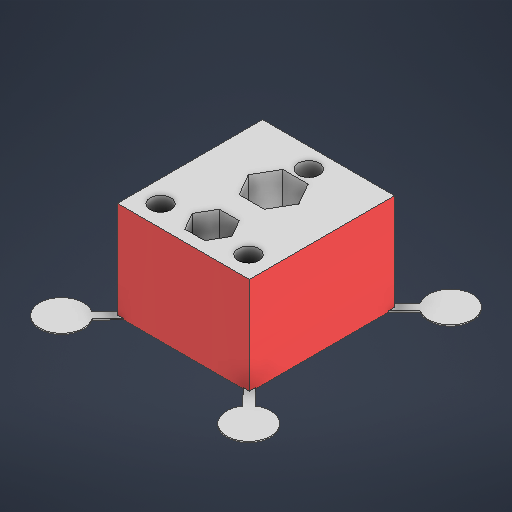
# Autodesk Inventor part: adapter-optical
Saved by Autodesk Inventor 2026.2 (Build 302298000, 298)
## iProperties
Created: 2026-05-22
Part Number: adapter-optical
Material: Generic
Document SubType Name: Modeling
Designer: mayhe
Density: 1 g/cm^3
Appearance: Default
Author: mayhe
Autodesk Inventor part; units mm, degrees
ref_plane "YZ Plane" through (0, 0, 0) normal (1, 0, 0) x (0, 1, 0)
ref_plane "XZ Plane" through (0, 0, 0) normal (0, 1, 0) x (-1, 0, 0)
ref_plane "XY Plane" through (0, 0, 0) normal (0, 0, 1) x (1, 0, 0)
sketch "Sketch1" plane through (0, 0, 0) normal (1, 0, 0) x (0, 1, 0)
  line L0 (11.125, 16.5) -> (-11.125, 16.5)
  line L1 (-11.125, 16.5) -> (-11.125, -16.5)
  line L2 (-11.125, -16.5) -> (11.125, -16.5)
  line L3 (11.125, -16.5) -> (11.125, 16.5)
  line L4 (11.125, 16.5) -> (-11.125, -16.5) construction
  line L5 (-11.125, 16.5) -> (11.125, -16.5) construction
  point P0 (0, 0)
  dimension "d0" = 22.25
  dimension "d1" = 33
  constraints: 12 end point, 2 midpoint, 2 parallel, 1 horizontal, 1 perpendicular
  measures "d0" distance of L2.end L1.end
  measures "d1" distance of L1.end L0.end
extrude "Extrusion1" add sketch "Sketch1" along normal mid plane 30
sketch "Sketch2" plane through (-15, -11.125, -16.5) normal (0, -1, 0) x (1, 0, 0)
  circle A0 centre (15, 4.5) radius 2.25
  line L0 (0, 0) -> (30, 0) projected
  circle A1 centre (25, 28.2) radius 2.25
  circle A2 centre (5, 28.2) radius 2.25
  point P0 (15, 16.5)
  dimension "d4" = 4.5
  dimension "d5" = 4.5
  dimension "d6" = 4.5
  dimension "d7" = 4.5
  dimension "d8" = 23.7
  dimension "d9" = 10
  dimension "d10" = 10
  constraints: 3 centre point, 1 horizontal alignment
  measures "d4" diameter of A0
  measures "d5" distance from line of L0 A0.centre
  measures "d6" diameter of A1
  measures "d7" diameter of A2
  measures "d8" vertical distance of A1.centre A0.centre
  measures "d9" horizontal distance of A0.centre A1.centre
  measures "d10" horizontal distance of A2.centre A0.centre
hole "Hole1" at (0, -11.125, -12) at (-10, -11.125, 11.7) at (10, -11.125, 11.7) direction (0, 1, 0) diameter 4.75 depth 22.25 tip angle 118 counterbore diameter 7.5 counterbore depth 3
sketch "Sketch4" plane through (-15, -11.125, -16.5) normal (0, -1, 0) x (1, 0, 0)
  circle A0 centre (15, 12.5) radius 2.0256
  circle A1 centre (15, 26.5) radius 2.1001
  line L0 (30, 33) -> (0, 33) projected
  point P0 (15, 16.5)
  point P1 (15, 33)
  dimension "d23" = 14
  dimension "d24" = 6.5
  constraints: 2 centre point, 1 midpoint
  measures "d23" distance of A1.centre A0.centre
  measures "d24" distance of point (15, 33) A1.centre
hole "Big Hole" at (0, -11.125, -4) direction (0, 1, 0) diameter 6.75 depth 22.25 tip angle 118
hole "Small Hole1" at (0, -11.125, 10) direction (0, 1, 0) diameter 5.75 depth 22.25 tip angle 118
sketch "Sketch5" plane through (-15, 11.125, 16.5) normal (0, 1, 0) x (1, 0, 0)
  circle A0 centre (15, 6.5) radius 2.875 projected
  circle A1 centre (15, 20.5) radius 3.375 projected
  circle A2 centre (15, 20.5) radius 4.975
  circle A3 centre (15, 6.5) radius 3.925
  line L0 (17.2661, 10.425) -> (19.5322, 6.5)
  line L1 (19.5322, 6.5) -> (17.2661, 2.575)
  line L2 (17.2661, 2.575) -> (12.7339, 2.575)
  line L3 (12.7339, 2.575) -> (10.4678, 6.5)
  line L4 (10.4678, 6.5) -> (12.7339, 10.425)
  line L5 (12.7339, 10.425) -> (17.2661, 10.425)
  line L6 (17.8723, 25.475) -> (20.7446, 20.5)
  line L7 (20.7446, 20.5) -> (17.8723, 15.525)
  line L8 (17.8723, 15.525) -> (12.1277, 15.525)
  line L9 (12.1277, 15.525) -> (9.2554, 20.5)
  line L10 (9.2554, 20.5) -> (12.1277, 25.475)
  line L11 (12.1277, 25.475) -> (17.8723, 25.475)
  point P0 (15, 16.5)
  point P1 (15, 10.425)
  point P2 (15, 25.475)
  dimension "d39" = 9.95
  dimension "d40" = 7.85
  constraints: 24 end point, 4 coincident, 2 midpoint, 2 vertical alignment, 30 other
extrude "Big nut seat" cut sketch "Sketch5" against normal blind 8.1168 contours A1 | A2 | A2 L6 L7 | A2 L11 L6 | L7 L8 A2 | A2 L10 L11 | L8 L9 A2 | A2 L9 L10
extrude "small nut seat" cut sketch "Sketch5" against normal blind 6.6168 contours A0 | A3 | A3 L0 L1 | A3 L5 L0 | L1 L2 A3 | A3 L4 L5 | L2 L3 A3 | A3 L3 L4
sketch "Sketch6" plane through (15, 11.125, -16.5) normal (0, 0, -1) x (-1, 0, 0)
  line L0 (2.368, -2.6371) -> (27.632, -2.6371) construction
  line L1 (27.632, -2.6371) -> (27.632, -19.6129) construction
  line L2 (27.632, -19.6129) -> (2.368, -19.6129) construction
  line L3 (2.368, -19.6129) -> (2.368, -2.6371) construction
  line L4 (12.625, 0) -> (17.375, 0) projected
  line L5 (15, 0) -> (15, -22.25)
  line L6 (17.875, -22.25) -> (12.125, -22.25) projected
  line L7 (30, 0) -> (0, 0) projected
  spline S0 degree 2 poles (10.4806, -3.0109) (10.4806, -3.7828) (9.6573, -4.6653) (8.942, -4.6653) knots 0 0 0 1 2 2 2
  spline S1 degree 2 poles (8.942, -4.6653) (8.2242, -4.6653) (7.406, -3.7725) (7.406, -3.0109) knots 0 0 0 1 2 2 2
  spline S2 degree 2 poles (7.406, -3.0109) (7.406, -2.2468) (8.2242, -1.3565) (8.942, -1.3565) knots 0 0 0 1 2 2 2
  spline S3 degree 2 poles (8.942, -1.3565) (9.6573, -1.3565) (10.4806, -2.2416) (10.4806, -3.0109) knots 0 0 0 1 2 2 2
  spline S4 degree 2 poles (9.6573, -3.0109) (9.6573, -2.7253) (9.5415, -2.3265) (9.4412, -2.2005) knots 0 0 0 1 2 2 2
  spline S5 degree 2 poles (9.4412, -2.2005) (9.3408, -2.0692) (9.0835, -1.956) (8.9446, -1.956) knots 0 0 0 1 2 2 2
  spline S6 degree 2 poles (8.9446, -1.956) (8.7979, -1.956) (8.5587, -2.0615) (8.448, -2.1953) knots 0 0 0 1 2 2 2
  spline S7 degree 2 poles (8.448, -2.1953) (8.3503, -2.3188) (8.2293, -2.7279) (8.2293, -3.0109) knots 0 0 0 1 2 2 2
  spline S8 degree 2 poles (8.2293, -3.0109) (8.2293, -3.3043) (8.3451, -3.6902) (8.4455, -3.8214) knots 0 0 0 1 2 2 2
  spline S9 degree 2 poles (8.4455, -3.8214) (8.5458, -3.9526) (8.8057, -4.0658) (8.9446, -4.0658) knots 0 0 0 1 2 2 2
  spline S10 degree 2 poles (8.9446, -4.0658) (9.0861, -4.0658) (9.3486, -3.9449) (9.4438, -3.8163) knots 0 0 0 1 2 2 2
  spline S11 degree 2 poles (9.4438, -3.8163) (9.5467, -3.6773) (9.6573, -3.3094) (9.6573, -3.0109) knots 0 0 0 1 2 2 2
  spline S12 degree 2 poles (13.2568, -3.3686) (13.2568, -3.9423) (12.6754, -4.6448) (12.2482, -4.6448) knots 0 0 0 1 2 2 2
  spline S13 degree 2 poles (12.2482, -4.6448) (12.0707, -4.6448) (11.8057, -4.565) (11.6565, -4.4775) knots 0 0 0 1 2 2 2
  line L8 (11.6565, -4.4775) -> (11.6565, -5.4758)
  line L9 (11.6565, -5.4758) -> (10.9103, -5.4758)
  line L10 (10.9103, -5.4758) -> (10.9103, -2.203)
  line L11 (10.9103, -2.203) -> (11.6565, -2.203)
  line L12 (11.6565, -2.203) -> (11.6565, -2.4552)
  spline S14 degree 2 poles (11.6565, -2.4552) (11.8211, -2.3137) (12.1608, -2.1387) (12.3846, -2.1387) knots 0 0 0 1 2 2 2
  spline S15 degree 2 poles (12.3846, -2.1387) (12.8014, -2.1387) (13.2568, -2.8) (13.2568, -3.3686) knots 0 0 0 1 2 2 2
  spline S16 degree 2 poles (12.4927, -3.384) (12.4927, -3.0341) (12.2766, -2.7202) (12.0501, -2.7202) knots 0 0 0 1 2 2 2
  spline S17 degree 2 poles (12.0501, -2.7202) (11.9498, -2.7202) (11.7517, -2.7845) (11.6565, -2.8488) knots 0 0 0 1 2 2 2
  line L13 (11.6565, -2.8488) -> (11.6565, -4.0504)
  spline S18 degree 2 poles (11.6565, -4.0504) (11.7157, -4.0761) (11.8597, -4.0967) (11.9575, -4.0967) knots 0 0 0 1 2 2 2
  spline S19 degree 2 poles (11.9575, -4.0967) (12.2277, -4.0967) (12.4927, -3.7417) (12.4927, -3.384) knots 0 0 0 1 2 2 2
  spline S20 degree 2 poles (14.5742, -4.6448) (14.1188, -4.6448) (13.702, -4.2691) (13.702, -3.842) knots 0 0 0 1 2 2 2
  line L14 (13.702, -3.842) -> (13.702, -2.7228)
  line L15 (13.702, -2.7228) -> (13.4164, -2.7228)
  line L16 (13.4164, -2.7228) -> (13.4164, -2.203)
  line L17 (13.4164, -2.203) -> (13.702, -2.203)
  line L18 (13.702, -2.203) -> (13.702, -1.5186)
  line L19 (13.702, -1.5186) -> (14.4481, -1.5186)
  line L20 (14.4481, -1.5186) -> (14.4481, -2.203)
  line L21 (14.4481, -2.203) -> (15.1685, -2.203)
  line L22 (15.1685, -2.203) -> (15.1685, -2.7228)
  line L23 (15.1685, -2.7228) -> (14.4481, -2.7228)
  line L24 (14.4481, -2.7228) -> (14.4481, -3.5744)
  spline S21 degree 2 poles (14.4481, -3.5744) (14.4481, -3.7005) (14.4533, -3.8883) (14.4841, -3.9629) knots 0 0 0 1 2 2 2
  spline S22 degree 2 poles (14.4841, -3.9629) (14.515, -4.0375) (14.6668, -4.125) (14.8109, -4.125) knots 0 0 0 1 2 2 2
  spline S23 degree 2 poles (14.8109, -4.125) (14.8726, -4.125) (15.0656, -4.0736) (15.1042, -4.053) knots 0 0 0 1 2 2 2
  line L25 (15.1042, -4.053) -> (15.1685, -4.053)
  line L26 (15.1685, -4.053) -> (15.1685, -4.5779)
  spline S24 degree 2 poles (15.1685, -4.5779) (15.0476, -4.6087) (14.7749, -4.6448) (14.5742, -4.6448) knots 0 0 0 1 2 2 2
  line L27 (16.2183, -4.5984) -> (15.4721, -4.5984)
  line L28 (15.4721, -4.5984) -> (15.4721, -2.203)
  line L29 (15.4721, -2.203) -> (16.2183, -2.203)
  line L30 (16.2183, -2.203) -> (16.2183, -4.5984)
  line L31 (16.2414, -1.8608) -> (15.4516, -1.8608)
  line L32 (15.4516, -1.8608) -> (15.4516, -1.2794)
  line L33 (15.4516, -1.2794) -> (16.2414, -1.2794)
  line L34 (16.2414, -1.2794) -> (16.2414, -1.8608)
  spline S25 degree 2 poles (17.9627, -4.6628) (17.6668, -4.6628) (17.1754, -4.5135) (16.9927, -4.3592) knots 0 0 0 1 2 2 2
  spline S26 degree 2 poles (16.9927, -4.3592) (16.8152, -4.2022) (16.6145, -3.7314) (16.6145, -3.4123) knots 0 0 0 1 2 2 2
  spline S27 degree 2 poles (16.6145, -3.4123) (16.6145, -3.0675) (16.8306, -2.5864) (17.0185, -2.432) knots 0 0 0 1 2 2 2
  spline S28 degree 2 poles (17.0185, -2.432) (17.196, -2.2828) (17.6797, -2.1387) (17.9421, -2.1387) knots 0 0 0 1 2 2 2
  spline S29 degree 2 poles (17.9421, -2.1387) (18.1403, -2.1387) (18.5365, -2.2313) (18.7372, -2.3317) knots 0 0 0 1 2 2 2
  line L35 (18.7372, -2.3317) -> (18.7372, -2.9698)
  line L36 (18.7372, -2.9698) -> (18.642, -2.9698)
  spline S30 degree 2 poles (18.642, -2.9698) (18.5957, -2.926) (18.467, -2.8231) (18.3898, -2.7819) knots 0 0 0 1 2 2 2
  spline S31 degree 2 poles (18.3898, -2.7819) (18.3075, -2.7356) (18.1042, -2.6739) (17.9782, -2.6739) knots 0 0 0 1 2 2 2
  spline S32 degree 2 poles (17.9782, -2.6739) (17.6926, -2.6739) (17.3787, -3.0727) (17.3787, -3.4123) knots 0 0 0 1 2 2 2
  spline S33 degree 2 poles (17.3787, -3.4123) (17.3787, -3.7725) (17.7132, -4.1276) (17.991, -4.1276) knots 0 0 0 1 2 2 2
  spline S34 degree 2 poles (17.991, -4.1276) (18.1325, -4.1276) (18.3435, -4.0633) (18.4207, -4.017) knots 0 0 0 1 2 2 2
  spline S35 degree 2 poles (18.4207, -4.017) (18.4953, -3.9732) (18.6034, -3.8754) (18.642, -3.8368) knots 0 0 0 1 2 2 2
  line L37 (18.642, -3.8368) -> (18.7372, -3.8368)
  line L38 (18.7372, -3.8368) -> (18.7372, -4.4775)
  spline S36 degree 2 poles (18.7372, -4.4775) (18.6729, -4.5058) (18.5056, -4.5779) (18.4181, -4.601) knots 0 0 0 1 2 2 2
  spline S37 degree 2 poles (18.4181, -4.601) (18.3101, -4.6319) (18.1197, -4.6628) (17.9627, -4.6628) knots 0 0 0 1 2 2 2
  spline S38 degree 2 poles (20.4122, -4.3437) (20.335, -4.408) (20.214, -4.511) (20.1111, -4.5624) knots 0 0 0 1 2 2 2
  spline S39 degree 2 poles (20.1111, -4.5624) (20.0108, -4.6113) (19.8204, -4.6628) (19.6506, -4.6628) knots 0 0 0 1 2 2 2
  spline S40 degree 2 poles (19.6506, -4.6628) (19.3315, -4.6628) (18.9121, -4.2357) (18.9121, -3.9115) knots 0 0 0 1 2 2 2
  spline S41 degree 2 poles (18.9121, -3.9115) (18.9121, -3.6465) (19.1257, -3.3171) (19.3264, -3.2219) knots 0 0 0 1 2 2 2
  spline S42 degree 2 poles (19.3264, -3.2219) (19.5296, -3.1241) (20.0931, -3.047) (20.4173, -3.0264) knots 0 0 0 1 2 2 2
  line L39 (20.4173, -3.0264) -> (20.4173, -3.0135)
  spline S43 degree 2 poles (20.4173, -3.0135) (20.4173, -2.8154) (20.124, -2.6636) (19.8307, -2.6636) knots 0 0 0 1 2 2 2
  spline S44 degree 2 poles (19.8307, -2.6636) (19.6995, -2.6636) (19.3444, -2.7588) (19.1772, -2.8334) knots 0 0 0 1 2 2 2
  line L40 (19.1772, -2.8334) -> (19.1128, -2.8334)
  line L41 (19.1128, -2.8334) -> (19.1128, -2.2545)
  spline S45 degree 2 poles (19.1128, -2.2545) (19.2235, -2.2236) (19.7175, -2.1361) (19.9696, -2.1361) knots 0 0 0 1 2 2 2
  spline S46 degree 2 poles (19.9696, -2.1361) (20.5871, -2.1361) (21.1532, -2.5478) (21.1532, -2.9698) knots 0 0 0 1 2 2 2
  line L42 (21.1532, -2.9698) -> (21.1532, -4.5984)
  line L43 (21.1532, -4.5984) -> (20.4122, -4.5984)
  line L44 (20.4122, -4.5984) -> (20.4122, -4.3437)
  line L45 (20.4122, -3.9732) -> (20.4122, -3.4766)
  spline S47 degree 2 poles (20.4122, -3.4766) (20.2218, -3.4946) (19.9876, -3.523) (19.8744, -3.5641) knots 0 0 0 1 2 2 2
  spline S48 degree 2 poles (19.8744, -3.5641) (19.7741, -3.5976) (19.666, -3.7365) (19.666, -3.8497) knots 0 0 0 1 2 2 2
  spline S49 degree 2 poles (19.666, -3.8497) (19.666, -4.017) (19.8487, -4.143) (20.0262, -4.143) knots 0 0 0 1 2 2 2
  spline S50 degree 2 poles (20.0262, -4.143) (20.124, -4.143) (20.3298, -4.053) (20.4122, -3.9732) knots 0 0 0 1 2 2 2
  line L46 (22.4525, -4.5984) -> (21.7064, -4.5984)
  line L47 (21.7064, -4.5984) -> (21.7064, -1.2819)
  line L48 (21.7064, -1.2819) -> (22.4525, -1.2819)
  line L49 (22.4525, -1.2819) -> (22.4525, -4.5984)
  spline S51 degree 2 poles (8.3014, -9.8877) (7.5861, -9.8877) (6.7473, -9.0232) (6.7473, -8.2411) knots 0 0 0 1 2 2 2
  spline S52 degree 2 poles (6.7473, -8.2411) (6.7473, -7.4872) (7.5887, -6.5892) (8.3039, -6.5892) knots 0 0 0 1 2 2 2
  spline S53 degree 2 poles (8.3039, -6.5892) (8.4918, -6.5892) (8.7954, -6.633) (8.9343, -6.669) knots 0 0 0 1 2 2 2
  spline S54 degree 2 poles (8.9343, -6.669) (9.0424, -6.7025) (9.2971, -6.8131) (9.3769, -6.8543) knots 0 0 0 1 2 2 2
  line L50 (9.3769, -6.8543) -> (9.3769, -7.6107)
  line L51 (9.3769, -7.6107) -> (9.2971, -7.6107)
  spline S55 degree 2 poles (9.2971, -7.6107) (9.2379, -7.5592) (9.063, -7.4152) (8.9523, -7.3483) knots 0 0 0 1 2 2 2
  spline S56 degree 2 poles (8.9523, -7.3483) (8.8417, -7.2788) (8.5767, -7.1836) (8.43, -7.1836) knots 0 0 0 1 2 2 2
  spline S57 degree 2 poles (8.43, -7.1836) (8.2576, -7.1836) (7.972, -7.2917) (7.8408, -7.428) knots 0 0 0 1 2 2 2
  spline S58 degree 2 poles (7.8408, -7.428) (7.7225, -7.5489) (7.5707, -7.9632) (7.5707, -8.2436) knots 0 0 0 1 2 2 2
  spline S59 degree 2 poles (7.5707, -8.2436) (7.5707, -8.5395) (7.7276, -8.9435) (7.8563, -9.067) knots 0 0 0 1 2 2 2
  spline S60 degree 2 poles (7.8563, -9.067) (7.9798, -9.1879) (8.2834, -9.2934) (8.4352, -9.2934) knots 0 0 0 1 2 2 2
  spline S61 degree 2 poles (8.4352, -9.2934) (8.5921, -9.2934) (8.8777, -9.1879) (8.9755, -9.1236) knots 0 0 0 1 2 2 2
  spline S62 degree 2 poles (8.9755, -9.1236) (9.0835, -9.0593) (9.2456, -8.9229) (9.3048, -8.8689) knots 0 0 0 1 2 2 2
  line L52 (9.3048, -8.8689) -> (9.3769, -8.8689)
  line L53 (9.3769, -8.8689) -> (9.3769, -9.615)
  spline S63 degree 2 poles (9.3769, -9.615) (9.2894, -9.6562) (9.0604, -9.7591) (8.9369, -9.7951) knots 0 0 0 1 2 2 2
  spline S64 degree 2 poles (8.9369, -9.7951) (8.7877, -9.8414) (8.5278, -9.8877) (8.3014, -9.8877) knots 0 0 0 1 2 2 2
  spline S65 degree 2 poles (11.1239, -9.5713) (11.0467, -9.6356) (10.9258, -9.7385) (10.8228, -9.79) knots 0 0 0 1 2 2 2
  spline S66 degree 2 poles (10.8228, -9.79) (10.7225, -9.8389) (10.5321, -9.8903) (10.3623, -9.8903) knots 0 0 0 1 2 2 2
  spline S67 degree 2 poles (10.3623, -9.8903) (10.0432, -9.8903) (9.6239, -9.4632) (9.6239, -9.139) knots 0 0 0 1 2 2 2
  spline S68 degree 2 poles (9.6239, -9.139) (9.6239, -8.874) (9.8374, -8.5447) (10.0381, -8.4495) knots 0 0 0 1 2 2 2
  spline S69 degree 2 poles (10.0381, -8.4495) (10.2414, -8.3517) (10.8048, -8.2745) (11.129, -8.2539) knots 0 0 0 1 2 2 2
  line L54 (11.129, -8.2539) -> (11.129, -8.2411)
  spline S70 degree 2 poles (11.129, -8.2411) (11.129, -8.0429) (10.8357, -7.8911) (10.5424, -7.8911) knots 0 0 0 1 2 2 2
  spline S71 degree 2 poles (10.5424, -7.8911) (10.4112, -7.8911) (10.0561, -7.9863) (9.8889, -8.061) knots 0 0 0 1 2 2 2
  line L55 (9.8889, -8.061) -> (9.8245, -8.061)
  line L56 (9.8245, -8.061) -> (9.8245, -7.482)
  spline S72 degree 2 poles (9.8245, -7.482) (9.9352, -7.4512) (10.4292, -7.3637) (10.6813, -7.3637) knots 0 0 0 1 2 2 2
  spline S73 degree 2 poles (10.6813, -7.3637) (11.2988, -7.3637) (11.8649, -7.7754) (11.8649, -8.1973) knots 0 0 0 1 2 2 2
  line L57 (11.8649, -8.1973) -> (11.8649, -9.826)
  line L58 (11.8649, -9.826) -> (11.1239, -9.826)
  line L59 (11.1239, -9.826) -> (11.1239, -9.5713)
  line L60 (11.1239, -9.2008) -> (11.1239, -8.7042)
  spline S74 degree 2 poles (11.1239, -8.7042) (10.9335, -8.7222) (10.6993, -8.7505) (10.5861, -8.7917) knots 0 0 0 1 2 2 2
  spline S75 degree 2 poles (10.5861, -8.7917) (10.4858, -8.8251) (10.3777, -8.9641) (10.3777, -9.0773) knots 0 0 0 1 2 2 2
  spline S76 degree 2 poles (10.3777, -9.0773) (10.3777, -9.2445) (10.5604, -9.3706) (10.7379, -9.3706) knots 0 0 0 1 2 2 2
  spline S77 degree 2 poles (10.7379, -9.3706) (10.8357, -9.3706) (11.0415, -9.2805) (11.1239, -9.2008) knots 0 0 0 1 2 2 2
  line L61 (15.2766, -9.826) -> (15.2766, -8.6296)
  spline S78 degree 2 poles (15.2766, -8.6296) (15.2766, -8.452) (15.2637, -8.2102) (15.2329, -8.133) knots 0 0 0 1 2 2 2
  spline S79 degree 2 poles (15.2329, -8.133) (15.1994, -8.0558) (15.0656, -7.9863) (14.9447, -7.9863) knots 0 0 0 1 2 2 2
  spline S80 degree 2 poles (14.9447, -7.9863) (14.8598, -7.9863) (14.6951, -8.061) (14.5973, -8.1304) knots 0 0 0 1 2 2 2
  line L62 (14.5973, -8.1304) -> (14.5973, -9.826)
  line L63 (14.5973, -9.826) -> (13.846, -9.826)
  line L64 (13.846, -9.826) -> (13.846, -8.6296)
  spline S81 degree 2 poles (13.846, -8.6296) (13.846, -8.4546) (13.8306, -8.2102) (13.7997, -8.133) knots 0 0 0 1 2 2 2
  spline S82 degree 2 poles (13.7997, -8.133) (13.7663, -8.0558) (13.6325, -7.9863) (13.5116, -7.9863) knots 0 0 0 1 2 2 2
  spline S83 degree 2 poles (13.5116, -7.9863) (13.4215, -7.9863) (13.244, -8.0713) (13.1616, -8.1304) knots 0 0 0 1 2 2 2
  line L65 (13.1616, -8.1304) -> (13.1616, -9.826)
  line L66 (13.1616, -9.826) -> (12.4155, -9.826)
  line L67 (12.4155, -9.826) -> (12.4155, -7.4306)
  line L68 (12.4155, -7.4306) -> (13.1616, -7.4306)
  line L69 (13.1616, -7.4306) -> (13.1616, -7.6956)
  spline S84 degree 2 poles (13.1616, -7.6956) (13.3443, -7.5412) (13.6711, -7.3663) (13.8743, -7.3663) knots 0 0 0 1 2 2 2
  spline S85 degree 2 poles (13.8743, -7.3663) (14.093, -7.3663) (14.4275, -7.5747) (14.515, -7.7831) knots 0 0 0 1 2 2 2
  spline S86 degree 2 poles (14.515, -7.7831) (14.7286, -7.5824) (15.1093, -7.3663) (15.3049, -7.3663) knots 0 0 0 1 2 2 2
  spline S87 degree 2 poles (15.3049, -7.3663) (15.4721, -7.3663) (15.7371, -7.4718) (15.8272, -7.5798) knots 0 0 0 1 2 2 2
  spline S88 degree 2 poles (15.8272, -7.5798) (15.9275, -7.6956) (16.0279, -8.0121) (16.0279, -8.2668) knots 0 0 0 1 2 2 2
  line L70 (16.0279, -8.2668) -> (16.0279, -9.826)
  line L71 (16.0279, -9.826) -> (15.2766, -9.826)
  spline S89 degree 2 poles (17.8084, -9.8903) (17.1291, -9.8903) (16.4061, -9.2419) (16.4061, -8.6424) knots 0 0 0 1 2 2 2
  spline S90 degree 2 poles (16.4061, -8.6424) (16.4061, -8.0558) (17.0802, -7.356) (17.6874, -7.356) knots 0 0 0 1 2 2 2
  spline S91 degree 2 poles (17.6874, -7.356) (18.2355, -7.356) (18.7912, -7.9503) (18.7912, -8.5009) knots 0 0 0 1 2 2 2
  line L72 (18.7912, -8.5009) -> (18.7912, -8.7711)
  line L73 (18.7912, -8.7711) -> (17.1523, -8.7711)
  spline S92 degree 2 poles (17.1523, -8.7711) (17.1626, -8.9383) (17.2835, -9.1596) (17.3812, -9.2265) knots 0 0 0 1 2 2 2
  spline S93 degree 2 poles (17.3812, -9.2265) (17.4764, -9.2934) (17.7337, -9.35) (17.8855, -9.35) knots 0 0 0 1 2 2 2
  spline S94 degree 2 poles (17.8855, -9.35) (18.0142, -9.35) (18.2663, -9.2934) (18.3718, -9.2445) knots 0 0 0 1 2 2 2
  spline S95 degree 2 poles (18.3718, -9.2445) (18.4645, -9.2059) (18.6188, -9.1107) (18.6677, -9.0747) knots 0 0 0 1 2 2 2
  line L74 (18.6677, -9.0747) -> (18.7475, -9.0747)
  line L75 (18.7475, -9.0747) -> (18.7475, -9.6922)
  spline S96 degree 2 poles (18.7475, -9.6922) (18.6549, -9.7282) (18.5056, -9.79) (18.3718, -9.8208) knots 0 0 0 1 2 2 2
  spline S97 degree 2 poles (18.3718, -9.8208) (18.2509, -9.8543) (17.9936, -9.8903) (17.8084, -9.8903) knots 0 0 0 1 2 2 2
  spline S98 degree 2 poles (18.0554, -8.3208) (18.0502, -8.0841) (17.8418, -7.8345) (17.6283, -7.8345) knots 0 0 0 1 2 2 2
  spline S99 degree 2 poles (17.6283, -7.8345) (17.4096, -7.8345) (17.1626, -8.097) (17.1497, -8.3208) knots 0 0 0 1 2 2 2
  line L76 (17.1497, -8.3208) -> (18.0554, -8.3208)
  line L77 (20.7827, -8.1381) -> (20.7209, -8.1381)
  spline S100 degree 2 poles (20.7209, -8.1381) (20.6772, -8.1227) (20.5151, -8.1073) (20.4173, -8.1073) knots 0 0 0 1 2 2 2
  spline S101 degree 2 poles (20.4173, -8.1073) (20.3015, -8.1073) (20.0417, -8.1767) (19.9207, -8.2231) knots 0 0 0 1 2 2 2
  line L78 (19.9207, -8.2231) -> (19.9207, -9.826)
  line L79 (19.9207, -9.826) -> (19.1746, -9.826)
  line L80 (19.1746, -9.826) -> (19.1746, -7.4306)
  line L81 (19.1746, -7.4306) -> (19.9207, -7.4306)
  line L82 (19.9207, -7.4306) -> (19.9207, -7.7754)
  spline S102 degree 2 poles (19.9207, -7.7754) (19.9722, -7.7291) (20.1523, -7.585) (20.2269, -7.5412) knots 0 0 0 1 2 2 2
  spline S103 degree 2 poles (20.2269, -7.5412) (20.3092, -7.4923) (20.5254, -7.4229) (20.6206, -7.4229) knots 0 0 0 1 2 2 2
  spline S104 degree 2 poles (20.6206, -7.4229) (20.6566, -7.4229) (20.7466, -7.428) (20.7827, -7.4306) knots 0 0 0 1 2 2 2
  line L83 (20.7827, -7.4306) -> (20.7827, -8.1381)
  spline S105 degree 2 poles (22.3882, -9.5713) (22.311, -9.6356) (22.1901, -9.7385) (22.0871, -9.79) knots 0 0 0 1 2 2 2
  spline S106 degree 2 poles (22.0871, -9.79) (21.9868, -9.8389) (21.7964, -9.8903) (21.6266, -9.8903) knots 0 0 0 1 2 2 2
  spline S107 degree 2 poles (21.6266, -9.8903) (21.3075, -9.8903) (20.8882, -9.4632) (20.8882, -9.139) knots 0 0 0 1 2 2 2
  spline S108 degree 2 poles (20.8882, -9.139) (20.8882, -8.874) (21.1017, -8.5447) (21.3024, -8.4495) knots 0 0 0 1 2 2 2
  spline S109 degree 2 poles (21.3024, -8.4495) (21.5057, -8.3517) (22.0691, -8.2745) (22.3933, -8.2539) knots 0 0 0 1 2 2 2
  line L84 (22.3933, -8.2539) -> (22.3933, -8.2411)
  spline S110 degree 2 poles (22.3933, -8.2411) (22.3933, -8.0429) (22.1, -7.8911) (21.8067, -7.8911) knots 0 0 0 1 2 2 2
  spline S111 degree 2 poles (21.8067, -7.8911) (21.6755, -7.8911) (21.3204, -7.9863) (21.1532, -8.061) knots 0 0 0 1 2 2 2
  line L85 (21.1532, -8.061) -> (21.0888, -8.061)
  line L86 (21.0888, -8.061) -> (21.0888, -7.482)
  spline S112 degree 2 poles (21.0888, -7.482) (21.1995, -7.4512) (21.6935, -7.3637) (21.9456, -7.3637) knots 0 0 0 1 2 2 2
  spline S113 degree 2 poles (21.9456, -7.3637) (22.5631, -7.3637) (23.1292, -7.7754) (23.1292, -8.1973) knots 0 0 0 1 2 2 2
  line L87 (23.1292, -8.1973) -> (23.1292, -9.826)
  line L88 (23.1292, -9.826) -> (22.3882, -9.826)
  line L89 (22.3882, -9.826) -> (22.3882, -9.5713)
  line L90 (22.3882, -9.2008) -> (22.3882, -8.7042)
  spline S114 degree 2 poles (22.3882, -8.7042) (22.1978, -8.7222) (21.9636, -8.7505) (21.8504, -8.7917) knots 0 0 0 1 2 2 2
  spline S115 degree 2 poles (21.8504, -8.7917) (21.7501, -8.8251) (21.642, -8.9641) (21.642, -9.0773) knots 0 0 0 1 2 2 2
  spline S116 degree 2 poles (21.642, -9.0773) (21.642, -9.2445) (21.8247, -9.3706) (22.0022, -9.3706) knots 0 0 0 1 2 2 2
  spline S117 degree 2 poles (22.0022, -9.3706) (22.1, -9.3706) (22.3058, -9.2805) (22.3882, -9.2008) knots 0 0 0 1 2 2 2
  line L91 (6.2868, -15.0535) -> (7.3597, -11.8785)
  line L92 (7.3597, -11.8785) -> (8.2293, -11.8785)
  line L93 (8.2293, -11.8785) -> (9.3022, -15.0535)
  line L94 (9.3022, -15.0535) -> (8.4815, -15.0535)
  line L95 (8.4815, -15.0535) -> (8.2834, -14.4052)
  line L96 (8.2834, -14.4052) -> (7.2851, -14.4052)
  line L97 (7.2851, -14.4052) -> (7.0844, -15.0535)
  line L98 (7.0844, -15.0535) -> (6.2868, -15.0535)
  line L99 (8.1084, -13.8288) -> (7.7842, -12.7791)
  line L100 (7.7842, -12.7791) -> (7.4574, -13.8288)
  line L101 (7.4574, -13.8288) -> (8.1084, -13.8288)
  line L102 (11.7517, -15.0535) -> (11.0055, -15.0535)
  line L103 (11.0055, -15.0535) -> (11.0055, -14.804)
  spline S118 degree 2 poles (11.0055, -14.804) (10.9335, -14.8631) (10.7482, -14.9995) (10.6762, -15.0355) knots 0 0 0 1 2 2 2
  spline S119 degree 2 poles (10.6762, -15.0355) (10.5887, -15.0767) (10.4137, -15.1204) (10.2928, -15.1204) knots 0 0 0 1 2 2 2
  spline S120 degree 2 poles (10.2928, -15.1204) (9.8837, -15.1204) (9.4052, -14.4412) (9.4052, -13.8751) knots 0 0 0 1 2 2 2
  spline S121 degree 2 poles (9.4052, -13.8751) (9.4052, -13.5612) (9.5673, -13.1007) (9.7088, -12.9309) knots 0 0 0 1 2 2 2
  spline S122 degree 2 poles (9.7088, -12.9309) (9.84, -12.7739) (10.2105, -12.5938) (10.4163, -12.5938) knots 0 0 0 1 2 2 2
  spline S123 degree 2 poles (10.4163, -12.5938) (10.6041, -12.5938) (10.846, -12.6736) (11.0055, -12.7559) knots 0 0 0 1 2 2 2
  line L104 (11.0055, -12.7559) -> (11.0055, -11.737)
  line L105 (11.0055, -11.737) -> (11.7517, -11.737)
  line L106 (11.7517, -11.737) -> (11.7517, -15.0535)
  line L107 (11.0055, -14.3949) -> (11.0055, -13.219)
  spline S124 degree 2 poles (11.0055, -13.219) (10.9515, -13.1907) (10.7714, -13.1547) (10.7071, -13.1547) knots 0 0 0 1 2 2 2
  spline S125 degree 2 poles (10.7071, -13.1547) (10.4395, -13.1547) (10.1693, -13.5304) (10.1693, -13.8674) knots 0 0 0 1 2 2 2
  spline S126 degree 2 poles (10.1693, -13.8674) (10.1693, -14.2225) (10.3854, -14.539) (10.6247, -14.539) knots 0 0 0 1 2 2 2
  spline S127 degree 2 poles (10.6247, -14.539) (10.7225, -14.539) (10.9232, -14.4618) (11.0055, -14.3949) knots 0 0 0 1 2 2 2
  spline S128 degree 2 poles (13.6428, -14.7988) (13.5656, -14.8631) (13.4447, -14.9661) (13.3417, -15.0175) knots 0 0 0 1 2 2 2
  spline S129 degree 2 poles (13.3417, -15.0175) (13.2414, -15.0664) (13.051, -15.1179) (12.8812, -15.1179) knots 0 0 0 1 2 2 2
  spline S130 degree 2 poles (12.8812, -15.1179) (12.5621, -15.1179) (12.1428, -14.6908) (12.1428, -14.3666) knots 0 0 0 1 2 2 2
  spline S131 degree 2 poles (12.1428, -14.3666) (12.1428, -14.1016) (12.3563, -13.7722) (12.557, -13.677) knots 0 0 0 1 2 2 2
  spline S132 degree 2 poles (12.557, -13.677) (12.7603, -13.5793) (13.3237, -13.5021) (13.6479, -13.4815) knots 0 0 0 1 2 2 2
  line L108 (13.6479, -13.4815) -> (13.6479, -13.4686)
  spline S133 degree 2 poles (13.6479, -13.4686) (13.6479, -13.2705) (13.3546, -13.1187) (13.0613, -13.1187) knots 0 0 0 1 2 2 2
  spline S134 degree 2 poles (13.0613, -13.1187) (12.9301, -13.1187) (12.575, -13.2139) (12.4078, -13.2885) knots 0 0 0 1 2 2 2
  line L109 (12.4078, -13.2885) -> (12.3434, -13.2885)
  line L110 (12.3434, -13.2885) -> (12.3434, -12.7096)
  spline S135 degree 2 poles (12.3434, -12.7096) (12.4541, -12.6787) (12.9481, -12.5912) (13.2002, -12.5912) knots 0 0 0 1 2 2 2
  spline S136 degree 2 poles (13.2002, -12.5912) (13.8177, -12.5912) (14.3838, -13.0029) (14.3838, -13.4249) knots 0 0 0 1 2 2 2
  line L111 (14.3838, -13.4249) -> (14.3838, -15.0535)
  line L112 (14.3838, -15.0535) -> (13.6428, -15.0535)
  line L113 (13.6428, -15.0535) -> (13.6428, -14.7988)
  line L114 (13.6428, -14.4283) -> (13.6428, -13.9317)
  spline S137 degree 2 poles (13.6428, -13.9317) (13.4524, -13.9498) (13.2182, -13.9781) (13.105, -14.0192) knots 0 0 0 1 2 2 2
  spline S138 degree 2 poles (13.105, -14.0192) (13.0047, -14.0527) (12.8966, -14.1916) (12.8966, -14.3048) knots 0 0 0 1 2 2 2
  spline S139 degree 2 poles (12.8966, -14.3048) (12.8966, -14.4721) (13.0793, -14.5981) (13.2568, -14.5981) knots 0 0 0 1 2 2 2
  spline S140 degree 2 poles (13.2568, -14.5981) (13.3546, -14.5981) (13.5604, -14.5081) (13.6428, -14.4283) knots 0 0 0 1 2 2 2
  spline S141 degree 2 poles (17.2835, -13.8237) (17.2835, -14.3974) (16.702, -15.0999) (16.2749, -15.0999) knots 0 0 0 1 2 2 2
  spline S142 degree 2 poles (16.2749, -15.0999) (16.0974, -15.0999) (15.8323, -15.0201) (15.6831, -14.9326) knots 0 0 0 1 2 2 2
  line L115 (15.6831, -14.9326) -> (15.6831, -15.9309)
  line L116 (15.6831, -15.9309) -> (14.937, -15.9309)
  line L117 (14.937, -15.9309) -> (14.937, -12.6581)
  line L118 (14.937, -12.6581) -> (15.6831, -12.6581)
  line L119 (15.6831, -12.6581) -> (15.6831, -12.9103)
  spline S143 degree 2 poles (15.6831, -12.9103) (15.8478, -12.7688) (16.1874, -12.5938) (16.4113, -12.5938) knots 0 0 0 1 2 2 2
  spline S144 degree 2 poles (16.4113, -12.5938) (16.8281, -12.5938) (17.2835, -13.2551) (17.2835, -13.8237) knots 0 0 0 1 2 2 2
  spline S145 degree 2 poles (16.5193, -13.8391) (16.5193, -13.4892) (16.3032, -13.1753) (16.0768, -13.1753) knots 0 0 0 1 2 2 2
  spline S146 degree 2 poles (16.0768, -13.1753) (15.9764, -13.1753) (15.7783, -13.2396) (15.6831, -13.304) knots 0 0 0 1 2 2 2
  line L120 (15.6831, -13.304) -> (15.6831, -14.5055)
  spline S147 degree 2 poles (15.6831, -14.5055) (15.7423, -14.5312) (15.8864, -14.5518) (15.9841, -14.5518) knots 0 0 0 1 2 2 2
  spline S148 degree 2 poles (15.9841, -14.5518) (16.2543, -14.5518) (16.5193, -14.1968) (16.5193, -13.8391) knots 0 0 0 1 2 2 2
  spline S149 degree 2 poles (18.6008, -15.0999) (18.1454, -15.0999) (17.7286, -14.7242) (17.7286, -14.2971) knots 0 0 0 1 2 2 2
  line L121 (17.7286, -14.2971) -> (17.7286, -13.1779)
  line L122 (17.7286, -13.1779) -> (17.443, -13.1779)
  line L123 (17.443, -13.1779) -> (17.443, -12.6581)
  line L124 (17.443, -12.6581) -> (17.7286, -12.6581)
  line L125 (17.7286, -12.6581) -> (17.7286, -11.9737)
  line L126 (17.7286, -11.9737) -> (18.4747, -11.9737)
  line L127 (18.4747, -11.9737) -> (18.4747, -12.6581)
  line L128 (18.4747, -12.6581) -> (19.1952, -12.6581)
  line L129 (19.1952, -12.6581) -> (19.1952, -13.1779)
  line L130 (19.1952, -13.1779) -> (18.4747, -13.1779)
  line L131 (18.4747, -13.1779) -> (18.4747, -14.0295)
  spline S150 degree 2 poles (18.4747, -14.0295) (18.4747, -14.1556) (18.4799, -14.3434) (18.5108, -14.418) knots 0 0 0 1 2 2 2
  spline S151 degree 2 poles (18.5108, -14.418) (18.5416, -14.4926) (18.6934, -14.5801) (18.8375, -14.5801) knots 0 0 0 1 2 2 2
  spline S152 degree 2 poles (18.8375, -14.5801) (18.8993, -14.5801) (19.0923, -14.5287) (19.1308, -14.5081) knots 0 0 0 1 2 2 2
  line L132 (19.1308, -14.5081) -> (19.1952, -14.5081)
  line L133 (19.1952, -14.5081) -> (19.1952, -15.033)
  spline S153 degree 2 poles (19.1952, -15.033) (19.0742, -15.0638) (18.8015, -15.0999) (18.6008, -15.0999) knots 0 0 0 1 2 2 2
  spline S154 degree 2 poles (20.7261, -15.1179) (20.0468, -15.1179) (19.3238, -14.4695) (19.3238, -13.87) knots 0 0 0 1 2 2 2
  spline S155 degree 2 poles (19.3238, -13.87) (19.3238, -13.2834) (19.9979, -12.5835) (20.6051, -12.5835) knots 0 0 0 1 2 2 2
  spline S156 degree 2 poles (20.6051, -12.5835) (21.1532, -12.5835) (21.7089, -13.1779) (21.7089, -13.7285) knots 0 0 0 1 2 2 2
  line L134 (21.7089, -13.7285) -> (21.7089, -13.9986)
  line L135 (21.7089, -13.9986) -> (20.07, -13.9986)
  spline S157 degree 2 poles (20.07, -13.9986) (20.0803, -14.1659) (20.2012, -14.3872) (20.299, -14.4541) knots 0 0 0 1 2 2 2
  spline S158 degree 2 poles (20.299, -14.4541) (20.3942, -14.5209) (20.6514, -14.5776) (20.8033, -14.5776) knots 0 0 0 1 2 2 2
  spline S159 degree 2 poles (20.8033, -14.5776) (20.9319, -14.5776) (21.184, -14.5209) (21.2895, -14.4721) knots 0 0 0 1 2 2 2
  spline S160 degree 2 poles (21.2895, -14.4721) (21.3822, -14.4335) (21.5365, -14.3383) (21.5854, -14.3022) knots 0 0 0 1 2 2 2
  line L136 (21.5854, -14.3022) -> (21.6652, -14.3022)
  line L137 (21.6652, -14.3022) -> (21.6652, -14.9198)
  spline S161 degree 2 poles (21.6652, -14.9198) (21.5726, -14.9558) (21.4233, -15.0175) (21.2895, -15.0484) knots 0 0 0 1 2 2 2
  spline S162 degree 2 poles (21.2895, -15.0484) (21.1686, -15.0818) (20.9113, -15.1179) (20.7261, -15.1179) knots 0 0 0 1 2 2 2
  spline S163 degree 2 poles (20.9731, -13.5484) (20.9679, -13.3117) (20.7595, -13.0621) (20.546, -13.0621) knots 0 0 0 1 2 2 2
  spline S164 degree 2 poles (20.546, -13.0621) (20.3273, -13.0621) (20.0803, -13.3245) (20.0674, -13.5484) knots 0 0 0 1 2 2 2
  line L138 (20.0674, -13.5484) -> (20.9731, -13.5484)
  line L139 (23.7004, -13.3657) -> (23.6386, -13.3657)
  spline S165 degree 2 poles (23.6386, -13.3657) (23.5949, -13.3503) (23.4328, -13.3348) (23.335, -13.3348) knots 0 0 0 1 2 2 2
  spline S166 degree 2 poles (23.335, -13.3348) (23.2192, -13.3348) (22.9594, -13.4043) (22.8384, -13.4506) knots 0 0 0 1 2 2 2
  line L140 (22.8384, -13.4506) -> (22.8384, -15.0535)
  line L141 (22.8384, -15.0535) -> (22.0923, -15.0535)
  line L142 (22.0923, -15.0535) -> (22.0923, -12.6581)
  line L143 (22.0923, -12.6581) -> (22.8384, -12.6581)
  line L144 (22.8384, -12.6581) -> (22.8384, -13.0029)
  spline S167 degree 2 poles (22.8384, -13.0029) (22.8899, -12.9566) (23.07, -12.8125) (23.1446, -12.7688) knots 0 0 0 1 2 2 2
  spline S168 degree 2 poles (23.1446, -12.7688) (23.227, -12.7199) (23.4431, -12.6504) (23.5383, -12.6504) knots 0 0 0 1 2 2 2
  spline S169 degree 2 poles (23.5383, -12.6504) (23.5743, -12.6504) (23.6644, -12.6556) (23.7004, -12.6581) knots 0 0 0 1 2 2 2
  line L145 (23.7004, -12.6581) -> (23.7004, -13.3657)
  spline S170 degree 2 poles (6.7743, -19.2005) (6.7743, -19.7022) (6.1388, -20.348) (5.5831, -20.348) knots 0 0 0 1 2 2 2
  spline S171 degree 2 poles (5.5831, -20.348) (5.3052, -20.348) (4.8704, -20.1885) (4.7186, -20.0315) knots 0 0 0 1 2 2 2
  spline S172 degree 2 poles (4.7186, -20.0315) (4.5385, -19.8488) (4.3455, -19.2699) (4.3455, -18.866) knots 0 0 0 1 2 2 2
  spline S173 degree 2 poles (4.3455, -18.866) (4.3455, -18.4492) (4.5256, -17.8008) (4.7288, -17.5512) knots 0 0 0 1 2 2 2
  spline S174 degree 2 poles (4.7288, -17.5512) (4.9218, -17.3145) (5.5496, -17.0469) (5.9793, -17.0469) knots 0 0 0 1 2 2 2
  spline S175 degree 2 poles (5.9793, -17.0469) (6.1362, -17.0469) (6.4501, -17.0881) (6.5067, -17.101) knots 0 0 0 1 2 2 2
  line L146 (6.5067, -17.101) -> (6.5067, -17.7236)
  line L147 (6.5067, -17.7236) -> (6.4501, -17.7236)
  spline S176 degree 2 poles (6.4501, -17.7236) (6.3935, -17.6953) (6.1362, -17.6258) (5.9716, -17.6258) knots 0 0 0 1 2 2 2
  spline S177 degree 2 poles (5.9716, -17.6258) (5.5985, -17.6258) (5.192, -18.0195) (5.1431, -18.3848) knots 0 0 0 1 2 2 2
  spline S178 degree 2 poles (5.1431, -18.3848) (5.3, -18.2845) (5.6217, -18.1661) (5.8249, -18.1661) knots 0 0 0 1 2 2 2
  spline S179 degree 2 poles (5.8249, -18.1661) (5.9973, -18.1661) (6.2983, -18.2588) (6.4141, -18.3463) knots 0 0 0 1 2 2 2
  spline S180 degree 2 poles (6.4141, -18.3463) (6.5788, -18.4723) (6.7743, -18.8814) (6.7743, -19.2005) knots 0 0 0 1 2 2 2
  spline S181 degree 2 poles (5.8455, -19.679) (5.9073, -19.6018) (5.9741, -19.4217) (5.9741, -19.2391) knots 0 0 0 1 2 2 2
  spline S182 degree 2 poles (5.9741, -19.2391) (5.9741, -19.0847) (5.897, -18.884) (5.8275, -18.8248) knots 0 0 0 1 2 2 2
  spline S183 degree 2 poles (5.8275, -18.8248) (5.7555, -18.7631) (5.5779, -18.7193) (5.4776, -18.7193) knots 0 0 0 1 2 2 2
  spline S184 degree 2 poles (5.4776, -18.7193) (5.3927, -18.7193) (5.2177, -18.7631) (5.1405, -18.7939) knots 0 0 0 1 2 2 2
  spline S185 degree 2 poles (5.1405, -18.7939) (5.1405, -18.8145) (5.1354, -18.9123) (5.1354, -18.9869) knots 0 0 0 1 2 2 2
  spline S186 degree 2 poles (5.1354, -18.9869) (5.1354, -19.2622) (5.2306, -19.5941) (5.3052, -19.679) knots 0 0 0 1 2 2 2
  spline S187 degree 2 poles (5.3052, -19.679) (5.3592, -19.7485) (5.5033, -19.8077) (5.5805, -19.8077) knots 0 0 0 1 2 2 2
  spline S188 degree 2 poles (5.5805, -19.8077) (5.6448, -19.8077) (5.794, -19.7434) (5.8455, -19.679) knots 0 0 0 1 2 2 2
  line L148 (9.0462, -16.9646) -> (7.7829, -20.9706)
  line L149 (7.7829, -20.9706) -> (7.1706, -20.9706)
  line L150 (7.1706, -20.9706) -> (8.4313, -16.9646)
  line L151 (8.4313, -16.9646) -> (9.0462, -16.9646)
  spline S189 degree 2 poles (12.0849, -19.3986) (12.0849, -19.6018) (11.9151, -19.9543) (11.753, -20.083) knots 0 0 0 1 2 2 2
  spline S190 degree 2 poles (11.753, -20.083) (11.5909, -20.2116) (11.1252, -20.3557) (10.8241, -20.3557) knots 0 0 0 1 2 2 2
  spline S191 degree 2 poles (10.8241, -20.3557) (10.5025, -20.3557) (10.0214, -20.2091) (9.867, -20.083) knots 0 0 0 1 2 2 2
  spline S192 degree 2 poles (9.867, -20.083) (9.7152, -19.9569) (9.5711, -19.6147) (9.5711, -19.4243) knots 0 0 0 1 2 2 2
  spline S193 degree 2 poles (9.5711, -19.4243) (9.5711, -19.1516) (9.8721, -18.7888) (10.1577, -18.6679) knots 0 0 0 1 2 2 2
  line L152 (10.1577, -18.6679) -> (10.1577, -18.655)
  spline S194 degree 2 poles (10.1577, -18.655) (9.8773, -18.5186) (9.656, -18.1301) (9.656, -17.8908) knots 0 0 0 1 2 2 2
  spline S195 degree 2 poles (9.656, -17.8908) (9.656, -17.7159) (9.8104, -17.4097) (9.9622, -17.2888) knots 0 0 0 1 2 2 2
  spline S196 degree 2 poles (9.9622, -17.2888) (10.1089, -17.173) (10.554, -17.0341) (10.8318, -17.0341) knots 0 0 0 1 2 2 2
  spline S197 degree 2 poles (10.8318, -17.0341) (11.1252, -17.0341) (11.5626, -17.1601) (11.7041, -17.263) knots 0 0 0 1 2 2 2
  spline S198 degree 2 poles (11.7041, -17.263) (11.8482, -17.366) (12.0025, -17.6644) (12.0025, -17.8368) knots 0 0 0 1 2 2 2
  spline S199 degree 2 poles (12.0025, -17.8368) (12.0025, -18.0632) (11.7401, -18.426) (11.4699, -18.5521) knots 0 0 0 1 2 2 2
  line L153 (11.4699, -18.5521) -> (11.4699, -18.5624)
  spline S200 degree 2 poles (11.4699, -18.5624) (11.7864, -18.691) (12.0849, -19.1078) (12.0849, -19.3986) knots 0 0 0 1 2 2 2
  spline S201 degree 2 poles (11.2975, -19.432) (11.2975, -19.2751) (11.1638, -19.1104) (10.9476, -19.0049) knots 0 0 0 1 2 2 2
  spline S202 degree 2 poles (10.9476, -19.0049) (10.8859, -18.9766) (10.6517, -18.8866) (10.5617, -18.848) knots 0 0 0 1 2 2 2
  spline S203 degree 2 poles (10.5617, -18.848) (10.4794, -18.9303) (10.3481, -19.1773) (10.3481, -19.324) knots 0 0 0 1 2 2 2
  spline S204 degree 2 poles (10.3481, -19.324) (10.3481, -19.5452) (10.6312, -19.8103) (10.8602, -19.8103) knots 0 0 0 1 2 2 2
  spline S205 degree 2 poles (10.8602, -19.8103) (10.9245, -19.8103) (11.084, -19.7691) (11.1457, -19.7279) knots 0 0 0 1 2 2 2
  spline S206 degree 2 poles (11.1457, -19.7279) (11.2152, -19.679) (11.2975, -19.5452) (11.2975, -19.432) knots 0 0 0 1 2 2 2
  spline S207 degree 2 poles (11.2281, -17.9294) (11.2281, -17.7673) (11.0145, -17.5744) (10.8318, -17.5744) knots 0 0 0 1 2 2 2
  spline S208 degree 2 poles (10.8318, -17.5744) (10.6569, -17.5744) (10.4433, -17.7493) (10.4433, -17.878) knots 0 0 0 1 2 2 2
  spline S209 degree 2 poles (10.4433, -17.878) (10.4433, -18.0041) (10.572, -18.161) (10.7083, -18.2253) knots 0 0 0 1 2 2 2
  spline S210 degree 2 poles (10.7083, -18.2253) (10.7675, -18.2562) (10.9322, -18.3205) (11.0686, -18.372) knots 0 0 0 1 2 2 2
  spline S211 degree 2 poles (11.0686, -18.372) (11.1509, -18.2639) (11.2281, -18.0607) (11.2281, -17.9294) knots 0 0 0 1 2 2 2
  line L154 (14.3465, -16.9646) -> (13.0832, -20.9706)
  line L155 (13.0832, -20.9706) -> (12.4708, -20.9706)
  line L156 (12.4708, -20.9706) -> (13.7315, -16.9646)
  line L157 (13.7315, -16.9646) -> (14.3465, -16.9646)
  line L158 (17.3928, -20.2811) -> (15.0592, -20.2811)
  line L159 (15.0592, -20.2811) -> (15.0592, -19.7639)
  spline S212 degree 2 poles (15.0592, -19.7639) (15.3551, -19.5272) (15.8285, -19.1104) (16.006, -18.9226) knots 0 0 0 1 2 2 2
  spline S213 degree 2 poles (16.006, -18.9226) (16.2402, -18.6782) (16.4486, -18.3051) (16.4486, -18.1095) knots 0 0 0 1 2 2 2
  spline S214 degree 2 poles (16.4486, -18.1095) (16.4486, -17.8883) (16.1835, -17.6516) (15.9468, -17.6516) knots 0 0 0 1 2 2 2
  spline S215 degree 2 poles (15.9468, -17.6516) (15.8259, -17.6516) (15.6098, -17.7107) (15.4991, -17.7571) knots 0 0 0 1 2 2 2
  spline S216 degree 2 poles (15.4991, -17.7571) (15.3911, -17.8059) (15.2367, -17.9089) (15.1981, -17.9346) knots 0 0 0 1 2 2 2
  line L160 (15.1981, -17.9346) -> (15.1364, -17.9346)
  line L161 (15.1364, -17.9346) -> (15.1364, -17.2425)
  spline S217 degree 2 poles (15.1364, -17.2425) (15.2702, -17.1781) (15.8413, -17.0443) (16.1064, -17.0443) knots 0 0 0 1 2 2 2
  spline S218 degree 2 poles (16.1064, -17.0443) (16.6724, -17.0443) (17.2539, -17.5486) (17.2539, -18.0041) knots 0 0 0 1 2 2 2
  spline S219 degree 2 poles (17.2539, -18.0041) (17.2539, -18.2845) (16.9889, -18.8248) (16.6827, -19.1336) knots 0 0 0 1 2 2 2
  spline S220 degree 2 poles (16.6827, -19.1336) (16.4897, -19.324) (16.1269, -19.6199) (16.0472, -19.6816) knots 0 0 0 1 2 2 2
  line L162 (16.0472, -19.6816) -> (17.3928, -19.6816)
  line L163 (17.3928, -19.6816) -> (17.3928, -20.2811)
  spline S221 degree 2 poles (20.133, -18.6936) (20.133, -19.1053) (20.0018, -19.7228) (19.8551, -19.9312) knots 0 0 0 1 2 2 2
  spline S222 degree 2 poles (19.8551, -19.9312) (19.711, -20.137) (19.2453, -20.348) (18.9109, -20.348) knots 0 0 0 1 2 2 2
  spline S223 degree 2 poles (18.9109, -20.348) (18.5738, -20.348) (18.1107, -20.137) (17.964, -19.926) knots 0 0 0 1 2 2 2
  spline S224 degree 2 poles (17.964, -19.926) (17.8174, -19.7176) (17.6861, -19.1053) (17.6861, -18.6936) knots 0 0 0 1 2 2 2
  spline S225 degree 2 poles (17.6861, -18.6936) (17.6861, -18.2716) (17.8174, -17.6747) (17.9666, -17.4586) knots 0 0 0 1 2 2 2
  spline S226 degree 2 poles (17.9666, -17.4586) (18.1158, -17.2476) (18.5867, -17.0418) (18.9109, -17.0418) knots 0 0 0 1 2 2 2
  spline S227 degree 2 poles (18.9109, -17.0418) (19.2531, -17.0418) (19.711, -17.2579) (19.8577, -17.4715) knots 0 0 0 1 2 2 2
  spline S228 degree 2 poles (19.8577, -17.4715) (20.0018, -17.6799) (20.133, -18.2948) (20.133, -18.6936) knots 0 0 0 1 2 2 2
  spline S229 degree 2 poles (19.3328, -18.6936) (19.3328, -18.1044) (19.1399, -17.6284) (18.9109, -17.6284) knots 0 0 0 1 2 2 2
  spline S230 degree 2 poles (18.9109, -17.6284) (18.6819, -17.6284) (18.4863, -18.1044) (18.4863, -18.6962) knots 0 0 0 1 2 2 2
  spline S231 degree 2 poles (18.4863, -18.6962) (18.4863, -19.2777) (18.6819, -19.7614) (18.9109, -19.7614) knots 0 0 0 1 2 2 2
  spline S232 degree 2 poles (18.9109, -19.7614) (19.1373, -19.7614) (19.3328, -19.2777) (19.3328, -18.6936) knots 0 0 0 1 2 2 2
  line L164 (22.9555, -20.2811) -> (20.6219, -20.2811)
  line L165 (20.6219, -20.2811) -> (20.6219, -19.7639)
  spline S233 degree 2 poles (20.6219, -19.7639) (20.9177, -19.5272) (21.3912, -19.1104) (21.5687, -18.9226) knots 0 0 0 1 2 2 2
  spline S234 degree 2 poles (21.5687, -18.9226) (21.8028, -18.6782) (22.0112, -18.3051) (22.0112, -18.1095) knots 0 0 0 1 2 2 2
  spline S235 degree 2 poles (22.0112, -18.1095) (22.0112, -17.8883) (21.7462, -17.6516) (21.5095, -17.6516) knots 0 0 0 1 2 2 2
  spline S236 degree 2 poles (21.5095, -17.6516) (21.3886, -17.6516) (21.1725, -17.7107) (21.0618, -17.7571) knots 0 0 0 1 2 2 2
  spline S237 degree 2 poles (21.0618, -17.7571) (20.9538, -17.8059) (20.7994, -17.9089) (20.7608, -17.9346) knots 0 0 0 1 2 2 2
  line L166 (20.7608, -17.9346) -> (20.699, -17.9346)
  line L167 (20.699, -17.9346) -> (20.699, -17.2425)
  spline S238 degree 2 poles (20.699, -17.2425) (20.8328, -17.1781) (21.404, -17.0443) (21.669, -17.0443) knots 0 0 0 1 2 2 2
  spline S239 degree 2 poles (21.669, -17.0443) (22.2351, -17.0443) (22.8166, -17.5486) (22.8166, -18.0041) knots 0 0 0 1 2 2 2
  spline S240 degree 2 poles (22.8166, -18.0041) (22.8166, -18.2845) (22.5516, -18.8248) (22.2454, -19.1336) knots 0 0 0 1 2 2 2
  spline S241 degree 2 poles (22.2454, -19.1336) (22.0524, -19.324) (21.6896, -19.6199) (21.6099, -19.6816) knots 0 0 0 1 2 2 2
  line L168 (21.6099, -19.6816) -> (22.9555, -19.6816)
  line L169 (22.9555, -19.6816) -> (22.9555, -20.2811)
  spline S242 degree 2 poles (25.7188, -19.2005) (25.7188, -19.7022) (25.0833, -20.348) (24.5276, -20.348) knots 0 0 0 1 2 2 2
  spline S243 degree 2 poles (24.5276, -20.348) (24.2497, -20.348) (23.8149, -20.1885) (23.6631, -20.0315) knots 0 0 0 1 2 2 2
  spline S244 degree 2 poles (23.6631, -20.0315) (23.483, -19.8488) (23.29, -19.2699) (23.29, -18.866) knots 0 0 0 1 2 2 2
  spline S245 degree 2 poles (23.29, -18.866) (23.29, -18.4492) (23.4701, -17.8008) (23.6734, -17.5512) knots 0 0 0 1 2 2 2
  spline S246 degree 2 poles (23.6734, -17.5512) (23.8663, -17.3145) (24.4941, -17.0469) (24.9238, -17.0469) knots 0 0 0 1 2 2 2
  spline S247 degree 2 poles (24.9238, -17.0469) (25.0808, -17.0469) (25.3947, -17.0881) (25.4513, -17.101) knots 0 0 0 1 2 2 2
  line L170 (25.4513, -17.101) -> (25.4513, -17.7236)
  line L171 (25.4513, -17.7236) -> (25.3947, -17.7236)
  spline S248 degree 2 poles (25.3947, -17.7236) (25.338, -17.6953) (25.0808, -17.6258) (24.9161, -17.6258) knots 0 0 0 1 2 2 2
  spline S249 degree 2 poles (24.9161, -17.6258) (24.543, -17.6258) (24.1365, -18.0195) (24.0876, -18.3848) knots 0 0 0 1 2 2 2
  spline S250 degree 2 poles (24.0876, -18.3848) (24.2446, -18.2845) (24.5662, -18.1661) (24.7694, -18.1661) knots 0 0 0 1 2 2 2
  spline S251 degree 2 poles (24.7694, -18.1661) (24.9418, -18.1661) (25.2428, -18.2588) (25.3586, -18.3463) knots 0 0 0 1 2 2 2
  spline S252 degree 2 poles (25.3586, -18.3463) (25.5233, -18.4723) (25.7188, -18.8814) (25.7188, -19.2005) knots 0 0 0 1 2 2 2
  spline S253 degree 2 poles (24.79, -19.679) (24.8518, -19.6018) (24.9187, -19.4217) (24.9187, -19.2391) knots 0 0 0 1 2 2 2
  spline S254 degree 2 poles (24.9187, -19.2391) (24.9187, -19.0847) (24.8415, -18.884) (24.772, -18.8248) knots 0 0 0 1 2 2 2
  spline S255 degree 2 poles (24.772, -18.8248) (24.7, -18.7631) (24.5224, -18.7193) (24.4221, -18.7193) knots 0 0 0 1 2 2 2
  spline S256 degree 2 poles (24.4221, -18.7193) (24.3372, -18.7193) (24.1622, -18.7631) (24.085, -18.7939) knots 0 0 0 1 2 2 2
  spline S257 degree 2 poles (24.085, -18.7939) (24.085, -18.8145) (24.0799, -18.9123) (24.0799, -18.9869) knots 0 0 0 1 2 2 2
  spline S258 degree 2 poles (24.0799, -18.9869) (24.0799, -19.2622) (24.1751, -19.5941) (24.2497, -19.679) knots 0 0 0 1 2 2 2
  spline S259 degree 2 poles (24.2497, -19.679) (24.3037, -19.7485) (24.4478, -19.8077) (24.525, -19.8077) knots 0 0 0 1 2 2 2
  spline S260 degree 2 poles (24.525, -19.8077) (24.5893, -19.8077) (24.7386, -19.7434) (24.79, -19.679) knots 0 0 0 1 2 2 2
  point P0 (15, -11.125)
  point P1 (27.632, -11.125)
  point P2 (15, -11.125)
  point P3 (15, -2.6371)
  point P4 (15, 0)
  dimension "d0" = 22.25
  dimension "d1" = 33
  constraints: 6 midpoint, 2 end point, 1 horizontal alignment, 1 vertical alignment, 2 other
extrude "Text" cut sketch "Sketch6" along normal mid plane 1 contours L21 L22 L23 L5 | L5 L23 L24 S21 S22 S23 S24 S20 L14 L15 L16 L17 L18 L19 L20 L21 | S23 L25 L26 S24 L5 | S86 S87 S88 L70 L71 L61 S78 S79 L5 | L5 S79 S80 L62 L63 L64 S81 S82 S83 L65 L66 L67 L68 L69 S84 S85 S86 | L118 L119 S143 S144 S141 S142 L115 L116 L5 | L5 L116 L117 L118 | S0 S1 S2 S3 | S12 S13 L8 L9 L10 L11 L12 S14 S15 | L27 L28 L29 L30 | L31 L32 L33 L34 | S25 S26 S27 S28 S29 L35 L36 S30 S31 S32 S33 S34 S35 L37 L38 S36 S37 | S38 S39 S40 S41 S42 L39 S43 S44 L40 L41 S45 S46 L42 L43 L44 | L46 L47 L48 L49 | S51 S52 S53 S54 L50 L51 S55 S56 S57 S58 S59 S60 S61 S62 L52 L53 S63 S64 | S65 S66 S67 S68 S69 L54 S70 S71 L55 L56 S72 S73 L57 L58 L59 | S89 S90 S91 L72 L73 S92 S93 S94 S95 L74 L75 S96 S97 | L77 S100 S101 L78 L79 L80 L81 L82 S102 S103 S104 L83 | S105 S106 S107 S108 S109 L84 S110 S111 L85 L86 S112 S113 L87 L88 L89 | L91 L92 L93 L94 L95 L96 L97 L98 | L102 L103 S118 S119 S120 S121 S122 S123 L104 L105 L106 | S128 S129 S130 S131 S132 L108 S133 S134 L109 L110 S135 S136 L111 L112 L113 | S149 L121 L122 L123 L124 L125 L126 L127 L128 L129 L130 L131 S150 S151 S152 L132 L133 S153 | S154 S155 S156 L134 L135 S157 S158 S159 S160 L136 L137 S161 S162 | L139 S165 S166 L140 L141 L142 L143 L144 S167 S168 S169 L145 | S170 S171 S172 S173 S174 S175 L146 L147 S176 S177 S178 S179 S180 | L148 L149 L150 L151 | S189 S190 S191 S192 S193 L152 S194 S195 S196 S197 S198 S199 L153 S200 | L154 L155 L156 L157 | L158 L159 S212 S213 S214 S215 S216 L160 L161 S217 S218 S219 S220 L162 L163 | S221 S222 S223 S224 S225 S226 S227 S228 | L164 L165 S233 S234 S235 S236 S237 L166 L167 S238 S239 S240 S241 L168 L169 | S242 S243 S244 S245 S246 S247 L170 L171 S248 S249 S250 S251 S252
sketch "Sketch7" plane through (-15, -11.125, -16.5) normal (0, -1, 0) x (1, 0, 0)
  line L0 (30, 0) -> (30, 33) projected
  line L1 (30, 1.4) -> (28.5717, 0)
  line L2 (28.5717, 0) -> (35.5717, -7.1414)
  line L3 (35.5717, -7.1414) -> (37, -5.7414)
  line L4 (37, -5.7414) -> (30, 1.4)
  line L5 (0, 0) -> (30, 0) projected
  circle A0 centre (36.2859, -6.4414) radius 5
  line L6 (15, 0) -> (15, 33)
  line L7 (30, 33) -> (0, 33) projected
  line L8 (30, 16.5) -> (0, 16.5)
  line L9 (0, 33) -> (0, 0) projected
  line L10 (0, 1.4) -> (1.4283, 0)
  line L11 (1.4283, 0) -> (-5.5717, -7.1414)
  line L12 (-5.5717, -7.1414) -> (-7, -5.7414)
  line L13 (-7, -5.7414) -> (0, 1.4)
  circle A1 centre (-6.2859, -6.4414) radius 5
  line L14 (30, 31.6) -> (28.5717, 33)
  line L15 (28.5717, 33) -> (35.5717, 40.1414)
  line L16 (35.5717, 40.1414) -> (37, 38.7414)
  line L17 (37, 38.7414) -> (30, 31.6)
  circle A2 centre (36.2859, 39.4414) radius 5
  line L18 (1.4283, 33) -> (-5.5717, 40.1414)
  line L19 (-7, 38.7414) -> (0, 31.6)
  circle A3 centre (-6.2859, 39.4414) radius 5
  line L20 (-5.5717, 40.1414) -> (-7, 38.7414)
  line L21 (0, 31.6) -> (1.4283, 33)
  point P0 (15, 16.5)
  point P1 (33.5707, 35.2429)
  point P2 (32.1424, 36.6429)
  point P3 (-2.1424, 36.6429)
  point P4 (-3.5707, 35.2429)
  point P5 (-3.5707, -2.2429)
  point P6 (-2.1424, -3.6429)
  point P7 (33.5707, -2.2429)
  point P8 (32.1424, -3.6429)
  dimension "d48" = 2
  dimension "d50" = 1.4
  dimension "d51" = 10
  dimension "d54" = 10
  constraints: 36 end point, 15 symmetric about line, 5 midpoint, 4 centre point, 2 parallel, 2 point on line, 1 perpendicular, 3 other
  measures "d48" distance of L1.start L1.end
  measures "d50" distance of L0.start L1.start
  measures "d51" diameter of A0
  measures "d54" distance of L3.end L1.start
extrude "Micky mouse ears" add sketch "Sketch7" against normal blind 0.25 contours L5 L1 L0 | L0 L4 A0 L2 L5 | A0 L2 L3 L4 | L4 L3 L2 A0 | L14 L7 L0 | L0 L7 L15 A2 L17 | L11 A1 L13 L9 L5 | L5 L9 L10 | A2 L15 L16 L17 | L17 L16 L15 A2 | A1 L13 L12 L11 | L11 L12 L13 A1 | L21 L9 L7 | L7 L9 L19 A3 L18 | A3 L19 L20 L18 | L18 L20 L19 A3
equation "\"d50\" = d49"
equation "\"d49\" = 1.4"
body "Solid1"
